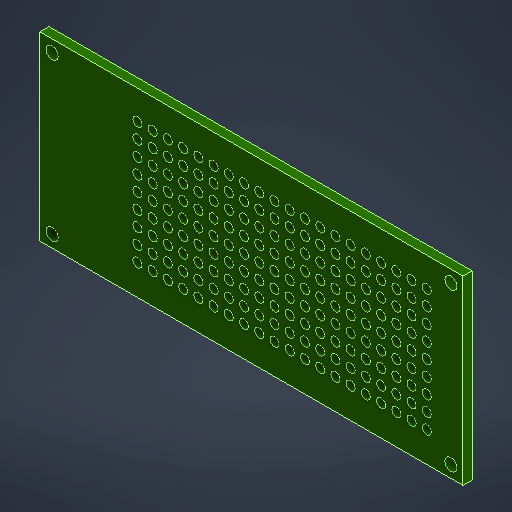
# Autodesk Inventor part: P_PCB_40x60
Saved by Autodesk Inventor 2026 (Build 300175000, 175)
## iProperties
Created: 2025-09-06
Part Number: P_PCB_40x60
Material: Generisch
Document SubType Name: Modeling
Designer: FAL
Density: 1 g/cm^3
Appearance: Vorgabe
Author: FAL
Autodesk Inventor part; units mm, degrees
ref_plane "YZ Plane" through (0, 0, 0) normal (1, 0, 0) x (0, 1, 0)
ref_plane "XZ Plane" through (0, 0, 0) normal (0, 1, 0) x (-1, 0, 0)
ref_plane "XY Plane" through (0, 0, 0) normal (0, 0, 1) x (1, 0, 0)
sketch "Skizze1" plane through (0, 0, 0) normal (0, 1, 0) x (-1, 0, 0)
  line L0 (-35, 15) -> (35, 15)
  line L1 (35, 15) -> (35, -15)
  line L2 (35, -15) -> (-35, -15)
  line L3 (-35, -15) -> (-35, 15)
  line L4 (-35, 15) -> (35, -15) construction
  line L5 (35, 15) -> (-35, -15) construction
  point P0 (0, 0)
  dimension "d0" = 30
  dimension "d1" = 70
  constraints: 12 end point, 2 midpoint, 2 parallel, 1 horizontal, 1 perpendicular
  measures "d0" distance between parallel lines of L2 L0
  measures "d1" distance of L1.end L2.end
extrude "Extrusion1" add sketch "Skizze1" along normal blind 1.5
sketch "Skizze2" plane through (0, 0, 0) normal (0, 1, 0) x (-1, 0, 0)
  line L0 (33, 13) -> (-33, 13) construction
  line L1 (-33, 13) -> (-33, -13) construction
  line L2 (-33, -13) -> (33, -13) construction
  line L3 (33, -13) -> (33, 13) construction
  line L4 (33, 13) -> (-33, -13) construction
  line L5 (-33, 13) -> (33, -13) construction
  circle A0 centre (-33, -13) radius 1
  circle A1 centre (-33, 13) radius 1
  circle A2 centre (33, 13) radius 1
  circle A3 centre (33, -13) radius 1
  point P0 (0, 0)
  dimension "d4" = 26
  dimension "d5" = 66
  dimension "d6" = 2
  constraints: 12 end point, 4 centre point, 4 coincident, 3 equal radius, 2 midpoint, 2 parallel, 1 horizontal, 1 perpendicular
  measures "d4" distance of L2.end L0.start
  measures "d5" distance of L1.end L2.end
  measures "d6" diameter of A0
extrude "Extrusion2" cut sketch "Skizze2" along normal blind 6
sketch "Skizze3" plane through (0, 0, 0) normal (0, 1, 0) x (-1, 0, 0)
  circle A0 centre (-29, -10) radius 0.75
  line L0 (-35, -15) -> (35, -15) projected
  line L1 (-35, 15) -> (-35, -15) projected
  circle A1 centre (-26.48, -10) radius 0.75
  circle A2 centre (-23.96, -10) radius 0.75
  circle A3 centre (-21.44, -10) radius 0.75
  circle A4 centre (-18.92, -10) radius 0.75
  circle A5 centre (-16.4, -10) radius 0.75
  circle A6 centre (-13.88, -10) radius 0.75
  circle A7 centre (-11.36, -10) radius 0.75
  circle A8 centre (-8.84, -10) radius 0.75
  circle A9 centre (-6.32, -10) radius 0.75
  circle A10 centre (-3.8, -10) radius 0.75
  circle A11 centre (-1.28, -10) radius 0.75
  circle A12 centre (1.24, -10) radius 0.75
  circle A13 centre (3.76, -10) radius 0.75
  circle A14 centre (6.28, -10) radius 0.75
  circle A15 centre (8.8, -10) radius 0.75
  circle A16 centre (11.32, -10) radius 0.75
  circle A17 centre (13.84, -10) radius 0.75
  circle A18 centre (16.36, -10) radius 0.75
  circle A19 centre (18.88, -10) radius 0.75
  circle A20 centre (-29, -7.48) radius 0.75
  circle A21 centre (-26.48, -7.48) radius 0.75
  circle A22 centre (-23.96, -7.48) radius 0.75
  circle A23 centre (-21.44, -7.48) radius 0.75
  circle A24 centre (-18.92, -7.48) radius 0.75
  circle A25 centre (-16.4, -7.48) radius 0.75
  circle A26 centre (-13.88, -7.48) radius 0.75
  circle A27 centre (-11.36, -7.48) radius 0.75
  circle A28 centre (-8.84, -7.48) radius 0.75
  circle A29 centre (-6.32, -7.48) radius 0.75
  circle A30 centre (-3.8, -7.48) radius 0.75
  circle A31 centre (-1.28, -7.48) radius 0.75
  circle A32 centre (1.24, -7.48) radius 0.75
  circle A33 centre (3.76, -7.48) radius 0.75
  circle A34 centre (6.28, -7.48) radius 0.75
  circle A35 centre (8.8, -7.48) radius 0.75
  circle A36 centre (11.32, -7.48) radius 0.75
  circle A37 centre (13.84, -7.48) radius 0.75
  circle A38 centre (16.36, -7.48) radius 0.75
  circle A39 centre (18.88, -7.48) radius 0.75
  circle A40 centre (-29, -4.96) radius 0.75
  circle A41 centre (-26.48, -4.96) radius 0.75
  circle A42 centre (-23.96, -4.96) radius 0.75
  circle A43 centre (-21.44, -4.96) radius 0.75
  circle A44 centre (-18.92, -4.96) radius 0.75
  circle A45 centre (-16.4, -4.96) radius 0.75
  circle A46 centre (-13.88, -4.96) radius 0.75
  circle A47 centre (-11.36, -4.96) radius 0.75
  circle A48 centre (-8.84, -4.96) radius 0.75
  circle A49 centre (-6.32, -4.96) radius 0.75
  circle A50 centre (-3.8, -4.96) radius 0.75
  circle A51 centre (-1.28, -4.96) radius 0.75
  circle A52 centre (1.24, -4.96) radius 0.75
  circle A53 centre (3.76, -4.96) radius 0.75
  circle A54 centre (6.28, -4.96) radius 0.75
  circle A55 centre (8.8, -4.96) radius 0.75
  circle A56 centre (11.32, -4.96) radius 0.75
  circle A57 centre (13.84, -4.96) radius 0.75
  circle A58 centre (16.36, -4.96) radius 0.75
  circle A59 centre (18.88, -4.96) radius 0.75
  circle A60 centre (-29, -2.44) radius 0.75
  circle A61 centre (-26.48, -2.44) radius 0.75
  circle A62 centre (-23.96, -2.44) radius 0.75
  circle A63 centre (-21.44, -2.44) radius 0.75
  circle A64 centre (-18.92, -2.44) radius 0.75
  circle A65 centre (-16.4, -2.44) radius 0.75
  circle A66 centre (-13.88, -2.44) radius 0.75
  circle A67 centre (-11.36, -2.44) radius 0.75
  circle A68 centre (-8.84, -2.44) radius 0.75
  circle A69 centre (-6.32, -2.44) radius 0.75
  circle A70 centre (-3.8, -2.44) radius 0.75
  circle A71 centre (-1.28, -2.44) radius 0.75
  circle A72 centre (1.24, -2.44) radius 0.75
  circle A73 centre (3.76, -2.44) radius 0.75
  circle A74 centre (6.28, -2.44) radius 0.75
  circle A75 centre (8.8, -2.44) radius 0.75
  circle A76 centre (11.32, -2.44) radius 0.75
  circle A77 centre (13.84, -2.44) radius 0.75
  circle A78 centre (16.36, -2.44) radius 0.75
  circle A79 centre (18.88, -2.44) radius 0.75
  circle A80 centre (-29, 0.08) radius 0.75
  circle A81 centre (-26.48, 0.08) radius 0.75
  circle A82 centre (-23.96, 0.08) radius 0.75
  circle A83 centre (-21.44, 0.08) radius 0.75
  circle A84 centre (-18.92, 0.08) radius 0.75
  circle A85 centre (-16.4, 0.08) radius 0.75
  circle A86 centre (-13.88, 0.08) radius 0.75
  circle A87 centre (-11.36, 0.08) radius 0.75
  circle A88 centre (-8.84, 0.08) radius 0.75
  circle A89 centre (-6.32, 0.08) radius 0.75
  circle A90 centre (-3.8, 0.08) radius 0.75
  circle A91 centre (-1.28, 0.08) radius 0.75
  circle A92 centre (1.24, 0.08) radius 0.75
  circle A93 centre (3.76, 0.08) radius 0.75
  circle A94 centre (6.28, 0.08) radius 0.75
  circle A95 centre (8.8, 0.08) radius 0.75
  circle A96 centre (11.32, 0.08) radius 0.75
  circle A97 centre (13.84, 0.08) radius 0.75
  circle A98 centre (16.36, 0.08) radius 0.75
  circle A99 centre (18.88, 0.08) radius 0.75
  circle A100 centre (-29, 2.6) radius 0.75
  circle A101 centre (-26.48, 2.6) radius 0.75
  circle A102 centre (-23.96, 2.6) radius 0.75
  circle A103 centre (-21.44, 2.6) radius 0.75
  circle A104 centre (-18.92, 2.6) radius 0.75
  circle A105 centre (-16.4, 2.6) radius 0.75
  circle A106 centre (-13.88, 2.6) radius 0.75
  circle A107 centre (-11.36, 2.6) radius 0.75
  circle A108 centre (-8.84, 2.6) radius 0.75
  circle A109 centre (-6.32, 2.6) radius 0.75
  circle A110 centre (-3.8, 2.6) radius 0.75
  circle A111 centre (-1.28, 2.6) radius 0.75
  circle A112 centre (1.24, 2.6) radius 0.75
  circle A113 centre (3.76, 2.6) radius 0.75
  circle A114 centre (6.28, 2.6) radius 0.75
  circle A115 centre (8.8, 2.6) radius 0.75
  circle A116 centre (11.32, 2.6) radius 0.75
  circle A117 centre (13.84, 2.6) radius 0.75
  circle A118 centre (16.36, 2.6) radius 0.75
  circle A119 centre (18.88, 2.6) radius 0.75
  circle A120 centre (-29, 5.12) radius 0.75
  circle A121 centre (-26.48, 5.12) radius 0.75
  circle A122 centre (-23.96, 5.12) radius 0.75
  circle A123 centre (-21.44, 5.12) radius 0.75
  circle A124 centre (-18.92, 5.12) radius 0.75
  circle A125 centre (-16.4, 5.12) radius 0.75
  circle A126 centre (-13.88, 5.12) radius 0.75
  circle A127 centre (-11.36, 5.12) radius 0.75
  circle A128 centre (-8.84, 5.12) radius 0.75
  circle A129 centre (-6.32, 5.12) radius 0.75
  circle A130 centre (-3.8, 5.12) radius 0.75
  circle A131 centre (-1.28, 5.12) radius 0.75
  circle A132 centre (1.24, 5.12) radius 0.75
  circle A133 centre (3.76, 5.12) radius 0.75
  circle A134 centre (6.28, 5.12) radius 0.75
  circle A135 centre (8.8, 5.12) radius 0.75
  circle A136 centre (11.32, 5.12) radius 0.75
  circle A137 centre (13.84, 5.12) radius 0.75
  circle A138 centre (16.36, 5.12) radius 0.75
  circle A139 centre (18.88, 5.12) radius 0.75
  circle A140 centre (-29, 7.64) radius 0.75
  circle A141 centre (-26.48, 7.64) radius 0.75
  circle A142 centre (-23.96, 7.64) radius 0.75
  circle A143 centre (-21.44, 7.64) radius 0.75
  circle A144 centre (-18.92, 7.64) radius 0.75
  circle A145 centre (-16.4, 7.64) radius 0.75
  circle A146 centre (-13.88, 7.64) radius 0.75
  circle A147 centre (-11.36, 7.64) radius 0.75
  circle A148 centre (-8.84, 7.64) radius 0.75
  circle A149 centre (-6.32, 7.64) radius 0.75
  circle A150 centre (-3.8, 7.64) radius 0.75
  circle A151 centre (-1.28, 7.64) radius 0.75
  circle A152 centre (1.24, 7.64) radius 0.75
  circle A153 centre (3.76, 7.64) radius 0.75
  circle A154 centre (6.28, 7.64) radius 0.75
  circle A155 centre (8.8, 7.64) radius 0.75
  circle A156 centre (11.32, 7.64) radius 0.75
  circle A157 centre (13.84, 7.64) radius 0.75
  circle A158 centre (16.36, 7.64) radius 0.75
  circle A159 centre (18.88, 7.64) radius 0.75
  circle A160 centre (-29, 10.16) radius 0.75
  circle A161 centre (-26.48, 10.16) radius 0.75
  circle A162 centre (-23.96, 10.16) radius 0.75
  circle A163 centre (-21.44, 10.16) radius 0.75
  circle A164 centre (-18.92, 10.16) radius 0.75
  circle A165 centre (-16.4, 10.16) radius 0.75
  circle A166 centre (-13.88, 10.16) radius 0.75
  circle A167 centre (-11.36, 10.16) radius 0.75
  circle A168 centre (-8.84, 10.16) radius 0.75
  circle A169 centre (-6.32, 10.16) radius 0.75
  circle A170 centre (-3.8, 10.16) radius 0.75
  circle A171 centre (-1.28, 10.16) radius 0.75
  circle A172 centre (1.24, 10.16) radius 0.75
  circle A173 centre (3.76, 10.16) radius 0.75
  circle A174 centre (6.28, 10.16) radius 0.75
  circle A175 centre (8.8, 10.16) radius 0.75
  circle A176 centre (11.32, 10.16) radius 0.75
  circle A177 centre (13.84, 10.16) radius 0.75
  circle A178 centre (16.36, 10.16) radius 0.75
  circle A179 centre (18.88, 10.16) radius 0.75
  circle A180 centre (21.4, -10) radius 0.75
  circle A181 centre (21.4, -7.48) radius 0.75
  circle A182 centre (21.4, -4.96) radius 0.75
  circle A183 centre (21.4, -2.44) radius 0.75
  circle A184 centre (21.4, 0.08) radius 0.75
  circle A185 centre (21.4, 2.6) radius 0.75
  circle A186 centre (21.4, 5.12) radius 0.75
  circle A187 centre (21.4, 7.64) radius 0.75
  circle A188 centre (21.4, 10.16) radius 0.75
  circle A189 centre (23.92, -10) radius 0.75
  circle A190 centre (23.92, -7.48) radius 0.75
  circle A191 centre (23.92, -4.96) radius 0.75
  circle A192 centre (23.92, -2.44) radius 0.75
  circle A193 centre (23.92, 0.08) radius 0.75
  circle A194 centre (23.92, 2.6) radius 0.75
  circle A195 centre (23.92, 5.12) radius 0.75
  circle A196 centre (23.92, 7.64) radius 0.75
  circle A197 centre (23.92, 10.16) radius 0.75
  circle A198 centre (26.44, -10) radius 0.75
  circle A199 centre (26.44, -7.48) radius 0.75
  circle A200 centre (26.44, -4.96) radius 0.75
  circle A201 centre (26.44, -2.44) radius 0.75
  circle A202 centre (26.44, 0.08) radius 0.75
  circle A203 centre (26.44, 2.6) radius 0.75
  circle A204 centre (26.44, 5.12) radius 0.75
  circle A205 centre (26.44, 7.64) radius 0.75
  circle A206 centre (26.44, 10.16) radius 0.75
  circle A207 centre (28.96, -10) radius 0.75
  circle A208 centre (28.96, -7.48) radius 0.75
  circle A209 centre (28.96, -4.96) radius 0.75
  circle A210 centre (28.96, -2.44) radius 0.75
  circle A211 centre (28.96, 0.08) radius 0.75
  circle A212 centre (28.96, 2.6) radius 0.75
  circle A213 centre (28.96, 5.12) radius 0.75
  circle A214 centre (28.96, 7.64) radius 0.75
  circle A215 centre (28.96, 10.16) radius 0.75
  point P0 (0, 0)
  dimension "d9" = 1.5
  dimension "d10" = 5
  dimension "d11" = 6
  dimension "d14" = 2.52
  dimension "d17" = 2.52
  constraints: 216 centre point, 1 horizontal, 1 vertical, 430 other
  measures "d9" diameter of A0
  measures "d10" distance from line of L0 A0.centre
  measures "d11" distance from line of L1 A0.centre
  measures "d14" distance of A0.centre A1.centre
  measures "d17" distance of A0.centre A20.centre
extrude "Extrusion3" cut sketch "Skizze3" along normal through all contours A0 | A1 | A2 | A3 | A4 | A5 | A6 | A7 | A8 | A9 | A10 | A11 | A12 | A13 | A14 | A15 | A16 | A17 | A18 | A19 | A20 | A21 | A22 | A23 | A24 | A25 | A26 | A27 | A28 | A29 | A30 | A31 | A32 | A33 | A34 | A35 | A36 | A37 | A38 | A39 | A40 | A41 | A42 | A43 | A44 | A45 | A46 | A47 | A48 | A49 | A50 | A51 | A52 | A53 | A54 | A55 | A56 | A57 | A58 | A59 | A60 | A61 | A62 | A63 | A64 | A65 | A66 | A67 | A68 | A69 | A70 | A71 | A72 | A73 | A74 | A75 | A76 | A77 | A78 | A79 | A80 | A81 | A82 | A83 | A84 | A85 | A86 | A87 | A88 | A89 | A90 | A91 | A92 | A93 | A94 | A95 | A96 | A97 | A98 | A99 | A100 | A101 | A102 | A103 | A104 | A105 | A106 | A107 | A108 | A109 | A110 | A111 | A112 | A113 | A114 | A115 | A116 | A117 | A118 | A119 | A120 | A121 | A122 | A123 | A124 | A125 | A126 | A127 | A128 | A129 | A130 | A131 | A132 | A133 | A134 | A135 | A136 | A137 | A138 | A139 | A140 | A141 | A142 | A143 | A144 | A145 | A146 | A147 | A148 | A149 | A150 | A151 | A152 | A153 | A154 | A155 | A156 | A157 | A158 | A159 | A160 | A161 | A162 | A163 | A164 | A165 | A166 | A167 | A168 | A169 | A170 | A171 | A172 | A173 | A174 | A175 | A176 | A177 | A178 | A179
